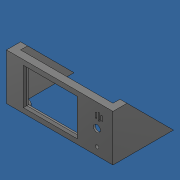
# Autodesk Inventor part: LCD_Holder
Saved by Autodesk Inventor 2020 (Build 240168000, 168)
## iProperties
Created: 2020-11-15
Part Number: LCD_Holder
Material: 一般
Document SubType Name: Modeling
Designer: kenta iguchi
Density: 1 g/cm^3
Appearance: 滑らか - 黒
Author: kenta iguchi
Autodesk Inventor part; units mm, degrees
ref_plane "YZ Plane" through (0, 0, 0) normal (1, 0, 0) x (0, 1, 0)
ref_plane "XZ Plane" through (0, 0, 0) normal (0, 1, 0) x (-1, 0, 0)
ref_plane "XY Plane" through (0, 0, 0) normal (0, 0, 1) x (1, 0, 0)
sketch "スケッチ1" plane through (0, 0, 0) normal (0, 0, 1) x (1, 0, 0)
  line L0 (18, -19) -> (-39.5, -19)
  line L1 (-39.5, -19) -> (-39.5, 19)
  line L2 (-39.5, 19) -> (18, 19)
  line L3 (18, 19) -> (18, -19)
  line L4 (18, -19) -> (-39.5, 19) construction
  line L5 (-39.5, -19) -> (18, 19) construction
  line L6 (-52.5, -23.5) -> (52.5, -23.5)
  line L7 (52.5, -23.5) -> (52.5, 23.5)
  line L8 (52.5, 23.5) -> (-52.5, 23.5)
  line L9 (-52.5, 23.5) -> (-52.5, -23.5)
  line L10 (-52.5, -23.5) -> (52.5, 23.5) construction
  line L11 (52.5, -23.5) -> (-52.5, 23.5) construction
  point P0 (0, 0)
  point P1 (0, 0)
  point P2 (-10.75, 0)
  point P3 (0, 0)
  dimension "d0" = 38
  dimension "d1" = 57.5
  dimension "d5" = 47
  dimension "d167" = 105
  dimension "d168" = 13
  constraints: 24 end point, 5 midpoint, 4 parallel, 2 horizontal, 2 perpendicular, 1 horizontal alignment, 1 other
  measures "d0" distance of L2.end L0.start
  measures "d1" distance of L0.start L0.end
  measures "d5" distance of L6.end L7.end
  measures "d167" distance of L6.start L6.end
  measures "d168" distance between parallel lines of L1 L9
extrude "押し出し1" add sketch "スケッチ1" against normal blind 4
sketch "スケッチ2" plane through (0, 0, 0) normal (0, 0, 1) x (1, 0, 0)
  line L0 (52.5, 23.5) -> (-52.5, 23.5) projected
  line L1 (-43.5, 20.5) -> (49.5, 20.5)
  line L2 (49.5, 20.5) -> (49.5, -20.5)
  line L3 (49.5, -20.5) -> (-43.5, -20.5)
  line L4 (-43.5, -20.5) -> (-43.5, 20.5)
  line L5 (-52.5, 23.5) -> (52.5, 23.5) projected
  line L6 (-52.5, 23.5) -> (-52.5, -23.5) projected
  point P0 (0, 0)
  point P1 (3, 20.5)
  dimension "d8" = 93
  dimension "d9" = 41
  dimension "d169" = 3
  dimension "d170" = 9
  constraints: 8 end point, 2 parallel, 1 horizontal, 1 midpoint, 1 perpendicular
  measures "d8" distance of L2.end L3.end
  measures "d9" distance of L1.end L2.end
  measures "d169" distance between parallel lines of L0 L1
  measures "d170" distance between parallel lines of L4 L6
hole "穴1" at (49.5, 20.5, 0) at (49.5, -20.5, 0) at (-43.5, -20.5, 0) at (-43.5, 20.5, 0) direction (0, 0, -1) diameter 4.3 depth 8 tip angle 118
sketch "スケッチ3" plane through (0, 0, 0) normal (0, 0, 1) x (1, 0, 0)
  line L0 (52.5, -23.5) -> (52.5, 23.5) projected
  circle A0 centre (42.65, -17.56) radius 2
  line L1 (-52.5, -23.5) -> (52.5, -23.5) projected
  point P0 (0, 0)
  dimension "d18" = 9.85
  dimension "d19" = 4
  dimension "d26" = 5.94
  constraints: 1 centre point, 1 coincident
  measures "d18" distance from line of point (42.65, -17.56) L0
  measures "d19" diameter of A0
  measures "d26" distance from line of point (42.65, -17.56) L1
extrude "押し出し2" cut sketch "スケッチ3" against normal blind 10
sketch "スケッチ4" plane through (0, 0, -4) normal (0, 0, -1) x (-1, 0, 0)
  circle A0 centre (-42.65, -17.56) radius 2 projected
  line L0 (-39.55, -14.46) -> (-45.75, -14.46)
  line L1 (-45.75, -14.46) -> (-45.75, -20.66)
  line L2 (-45.75, -20.66) -> (-39.55, -20.66)
  line L3 (-39.55, -20.66) -> (-39.55, -14.46)
  line L4 (-39.55, -14.46) -> (-45.75, -20.66) construction
  line L5 (-45.75, -14.46) -> (-39.55, -20.66) construction
  point P0 (0, 0)
  dimension "d22" = 6.2
  dimension "d23" = 6.2
  constraints: 12 end point, 2 midpoint, 2 parallel, 1 horizontal, 1 perpendicular
  measures "d22" distance of L2.end L1.end
  measures "d23" distance of L1.end L0.end
extrude "押し出し3" cut sketch "スケッチ4" against normal blind 1
sketch "スケッチ5" plane through (0, 0, 0) normal (0, 0, 1) x (1, 0, 0)
  circle A0 centre (42.37, 0.44) radius 4
  circle A1 centre (42.65, -17.56) radius 2 projected
  point P0 (0, 0)
  dimension "d29" = 8
  dimension "d171" = 18
  dimension "d172" = 0.28
  constraints: 1 centre point, 1 coincident
  measures "d29" diameter of A0
  measures "d171" vertical distance of A0.centre A1.centre
  measures "d172" horizontal distance of A1.centre A0.centre
extrude "押し出し4" cut sketch "スケッチ5" against normal through all contours A0
chamfer "面取り1" distance 2 angle 45 4 edges at (-39.5, 0, 0) (-10.75, 19, 0) (18, 0, 0) (-10.75, -19, 0)
sketch "スケッチ6" plane through (0, 0, -4) normal (0, 0, -1) x (-1, 0, 0)
  circle A0 centre (-42.37, 0.44) radius 4 projected
  line L0 (-48.87, -6.06) -> (-35.87, -6.06)
  line L1 (-35.87, -6.06) -> (-35.87, 6.94)
  line L2 (-35.87, 6.94) -> (-48.87, 6.94)
  line L3 (-48.87, 6.94) -> (-48.87, -6.06)
  line L4 (-48.87, -6.06) -> (-35.87, 6.94) construction
  line L5 (-35.87, -6.06) -> (-48.87, 6.94) construction
  point P0 (0, 0)
  dimension "d35" = 13
  dimension "d36" = 13
  constraints: 12 end point, 2 midpoint, 2 parallel, 1 horizontal, 1 perpendicular
  measures "d35" distance of L2.end L1.end
  measures "d36" distance of L1.end L0.end
extrude "押し出し5" cut sketch "スケッチ6" against normal blind 2
sketch "スケッチ7" plane through (0, 0, 0) normal (0, 0, 1) x (1, 0, 0)
  line L0 (52.5, 23.5) -> (-52.5, 23.5) projected
  line L1 (52.5, -23.5) -> (52.5, 23.5) projected
  circle A0 centre (44.69, 12.91) radius 4.5
  line L2 (44.69, 17.41) -> (44.69, 8.41) construction
  line L3 (43.94, 16.66) -> (43.94, 9.16)
  line L4 (45.44, 9.16) -> (45.44, 16.66)
  arc A1 (45.44, 16.66) -> (43.94, 16.66) centre (44.69, 16.66) ccw
  arc A2 (43.94, 9.16) -> (45.44, 9.16) centre (44.69, 9.16) ccw
  line L5 (41.69, 16.2641) -> (41.69, 9.5559) construction
  line L6 (40.94, 15.5141) -> (40.94, 10.3059)
  line L7 (42.44, 10.3059) -> (42.44, 15.5141)
  arc A3 (42.44, 15.5141) -> (40.94, 15.5141) centre (41.69, 15.5141) ccw
  arc A4 (40.94, 10.3059) -> (42.44, 10.3059) centre (41.69, 10.3059) ccw
  line L8 (47.69, 16.2641) -> (47.69, 9.5559) construction
  line L9 (46.94, 15.5141) -> (46.94, 10.3059)
  line L10 (48.44, 10.3059) -> (48.44, 15.5141)
  arc A5 (48.44, 15.5141) -> (46.94, 15.5141) centre (47.69, 15.5141) ccw
  arc A6 (46.94, 10.3059) -> (48.44, 10.3059) centre (47.69, 10.3059) ccw
  point P0 (0, 0)
  point P1 (41.69, 12.91)
  point P2 (47.69, 12.91)
  dimension "d39" = 7.81
  dimension "d40" = 10.59
  dimension "d41" = 9
  dimension "d42" = 1.5
  dimension "d43" = 1.5
  dimension "d44" = 1.5
  dimension "d45" = 3
  dimension "d46" = 6
  constraints: 24 end point, 24 point on circle, 12 tangent, 7 centre point, 6 point on line, 4 parallel, 3 midpoint, 2 coincident, 2 vertical
  measures "d39" distance from line of point (44.69, 12.91) L1
  measures "d40" distance from line of point (44.69, 12.91) L0
  measures "d41" diameter of A0
  measures "d42" diameter of A2
  measures "d43" diameter of A4
  measures "d44" diameter of A6
  measures "d45" distance of A0.centre point (41.69, 12.91)
  measures "d46" distance between parallel lines of L8 L5
extrude "押し出し6" cut sketch "スケッチ7" against normal blind 10 contours L10 A0 A6 L9 A5 | A0 A5 L10 | L10 A6 A0 | A1 L4 A2 L3 | A3 L7 A4 A0 L6 | A0 L6 A3 | A4 L6 A0
sketch "スケッチ8" plane through (0, 0, -4) normal (0, 0, -1) x (-1, 0, 0)
  line L0 (-46.94, 15.5141) -> (-46.94, 10.3059) projected
  arc A0 (-48.44, 10.3059) -> (-46.94, 10.3059) centre (-47.69, 10.3059) ccw projected
  line L1 (-48.44, 10.3059) -> (-48.44, 15.5141) projected
  arc A1 (-46.94, 15.5141) -> (-48.44, 15.5141) centre (-47.69, 15.5141) ccw projected
  line L2 (-45.44, 9.16) -> (-45.44, 16.66) projected
  arc A2 (-43.94, 16.66) -> (-45.44, 16.66) centre (-44.69, 16.66) ccw projected
  line L3 (-43.94, 16.66) -> (-43.94, 9.16) projected
  arc A3 (-45.44, 9.16) -> (-43.94, 9.16) centre (-44.69, 9.16) ccw projected
  line L4 (-40.94, 15.5141) -> (-40.94, 10.3059) projected
  arc A4 (-42.44, 10.3059) -> (-40.94, 10.3059) centre (-41.69, 10.3059) ccw projected
  line L5 (-42.44, 10.3059) -> (-42.44, 15.5141) projected
  arc A5 (-40.94, 15.5141) -> (-42.44, 15.5141) centre (-41.69, 15.5141) ccw projected
  line L6 (-44.69, 9.16) -> (-44.69, 16.66)
  circle A6 centre (-44.69, 12.91) radius 5
  point P0 (0, 0)
  dimension "d49" = 10
  constraints: 2 end point, 1 centre point, 1 coincident, 1 midpoint, 1 vertical
  measures "d49" diameter of A6
extrude "押し出し7" cut sketch "スケッチ8" against normal blind 2
sketch "スケッチ9" plane through (0, 0, 0) normal (0, 0, 1) x (1, 0, 0)
  line L0 (52.5, 23.5) -> (-52.5, 23.5) projected
  line L1 (-52.5, 23.5) -> (-52.5, -23.5) projected
  line L2 (-52.5, -23.5) -> (52.5, -23.5) projected
  line L3 (52.5, -23.5) -> (52.5, 23.5) projected
  line L4 (-55.5, 26.5) -> (55.5, 26.5)
  line L5 (55.5, 26.5) -> (55.5, -26.5)
  line L6 (55.5, -26.5) -> (-55.5, -26.5)
  line L7 (-55.5, -26.5) -> (-55.5, 26.5)
  circle A0 centre (49.5, 20.5) radius 2.15 projected
  circle A1 centre (49.5, 20.5) radius 4
  point P0 (0, 0)
  dimension "d52" = 3
  dimension "d67" = 8
  constraints: 8 end point, 1 centre point, 1 coincident, 3 other
  measures "d52" distance between parallel lines of L0 L4
  measures "d67" diameter of A1
extrude "押し出し8" add sketch "スケッチ9" against normal up to surface (4 mm away) contours L0 A1 | A1 L3 | L4 L5 L6 L7
sketch "スケッチ10" plane through (0, 0, -4) normal (0, 0, -1) x (-1, 0, 0)
  circle A0 centre (43.5, -20.5) radius 2.15 projected
  circle A1 centre (-49.5, 20.5) radius 2.15 projected
  circle A2 centre (43.5, 20.5) radius 2.15 projected
  circle A3 centre (-49.5, 20.5) radius 2.2
  circle A4 centre (43.5, 20.5) radius 2.2
  circle A5 centre (43.5, -20.5) radius 2.2
  circle A6 centre (-49.5, -20.5) radius 2.15 projected
  circle A7 centre (-49.5, -20.5) radius 2.2
  circle A8 centre (-49.5, 20.5) radius 2.15 projected
  circle A9 centre (-49.5, 20.5) radius 4
  circle A10 centre (43.5, 20.5) radius 4
  circle A11 centre (43.5, -20.5) radius 4
  circle A12 centre (-49.5, -20.5) radius 4
  point P0 (0, 0)
  dimension "d55" = 4.4
  dimension "d56" = 4.4
  dimension "d57" = 4.4
  dimension "d58" = 4.4
  dimension "d59" = 8
  dimension "d60" = 8
  dimension "d61" = 8
  dimension "d62" = 8
  constraints: 8 centre point, 8 coincident
  measures "d55" diameter of A3
  measures "d56" diameter of A4
  measures "d57" diameter of A5
  measures "d58" diameter of A7
  measures "d59" diameter of A9
  measures "d60" diameter of A10
  measures "d61" diameter of A11
  measures "d62" diameter of A12
extrude "押し出し9" add sketch "スケッチ10" along normal blind 3 contours A3 | A4 | A5 | A7 | A9 | A10 | A11 | A12
sketch "スケッチ11" plane through (0, 0, 0) normal (0, 0, 1) x (1, 0, 0)
  circle A0 centre (49.5, -20.5) radius 2.15 projected
  circle A1 centre (49.5, 20.5) radius 2.15 projected
  circle A2 centre (-43.5, -20.5) radius 2.15 projected
  circle A3 centre (-43.5, 20.5) radius 2.15 projected
  point P0 (0, 0)
extrude "押し出し10" add sketch "スケッチ11" against normal up to surface (4 mm away)
sketch "スケッチ12" plane through (0, 0, -4) normal (0, 0, -1) x (-1, 0, 0)
  circle A0 centre (43.5, 20.5) radius 4 projected
  arc A1 (-47.1508, 17.2625) -> (-47.5753, 16.9935) centre (-49.5, 20.5) ccw projected
  circle A2 centre (43.5, -20.5) radius 4 projected
  arc A3 (-45.75, -19.1081) -> (-45.5032, -20.66) centre (-49.5, -20.5) ccw projected
  line L0 (55.5, 26.5) -> (55.5, -26.5) projected
  line L1 (-55.5, 26.5) -> (55.5, 26.5) projected
  line L2 (-55.5, -26.5) -> (-55.5, 26.5) projected
  line L3 (55.5, -26.5) -> (-55.5, -26.5) projected
  line L4 (52.7, 23.7) -> (52.7, -23.7)
  line L5 (52.7, -23.7) -> (-52.7, -23.7)
  line L6 (-52.7, -23.7) -> (-52.7, 23.7)
  line L7 (-52.7, 23.7) -> (52.7, 23.7)
  circle A4 centre (-49.5, 20.5) radius 4 projected
  line L8 (-18, -19) -> (-18, 19) projected
  line L9 (-18, 19) -> (39.5, 19) projected
  line L10 (39.5, 19) -> (39.5, -19) projected
  line L11 (39.5, -19) -> (-18, -19) projected
  line L12 (-35.87, 6.94) -> (-35.87, -6.06) projected
  line L13 (-35.87, -6.06) -> (-48.87, -6.06) projected
  line L14 (-48.87, -6.06) -> (-48.87, 6.94) projected
  line L15 (-48.87, 6.94) -> (-35.87, 6.94) projected
  arc A5 (-47.1508, 17.2625) -> (-47.5753, 16.9935) centre (-49.5, 20.5) ccw projected
  arc A6 (-47.5753, 16.9935) -> (-47.1508, 17.2625) centre (-44.69, 12.91) ccw projected
  line L16 (55.5, -26.5) -> (-55.5, -26.5) projected
  line L17 (55.5, 26.5) -> (55.5, -26.5) projected
  line L18 (-55.5, 26.5) -> (55.5, 26.5) projected
  line L19 (-55.5, -26.5) -> (-55.5, 26.5) projected
  circle A7 centre (43.5, -20.5) radius 4 projected
  circle A8 centre (43.5, 20.5) radius 4 projected
  arc A9 (-45.75, -19.1081) -> (-45.5032, -20.66) centre (-49.5, -20.5) ccw projected
  line L20 (-45.75, -19.1081) -> (-45.75, -14.46) projected
  line L21 (-45.75, -14.46) -> (-39.55, -14.46) projected
  line L22 (-39.55, -14.46) -> (-39.55, -20.66) projected
  line L23 (-39.55, -20.66) -> (-45.5032, -20.66) projected
  point P0 (0, 0)
  point P1 (-47.1, 23.7)
  point P2 (41.1, 23.7)
  point P3 (52.7, 17.5876)
  point P4 (52.7, -17.5876)
  point P5 (41.1, -23.7)
  point P6 (-47.1, -23.7)
  point P7 (-52.7, -18.1)
  point P8 (-52.7, 18.1)
  point P9 (45.9, 23.7)
  point P10 (-51.9, 23.7)
  point P11 (-52.7, 22.9)
  point P12 (-52.7, -22.9)
  point P13 (-51.9, -23.7)
  point P14 (45.9, -23.7)
  dimension "d68" = 2.8
  constraints: 8 end point, 3 other
  measures "d68" distance between parallel lines of L1 L7
extrude "押し出し11" add sketch "スケッチ12" along normal blind 4 contours A1 L6 L7 | L5 L6 A3 | L0 L3 L2 L1
sketch "スケッチ14" plane through (0, 0, -8) normal (0, 0, -1) x (-1, 0, 0)
  line L0 (55.5, -26.5) -> (55.5, 26.5) projected
  line L1 (-52.7, -18.1) -> (-52.7, 18.1) projected
  line L2 (52.7, 23.7) -> (52.7, -23.7) projected
  line L3 (-55.5, 26.5) -> (55.5, 26.5) projected
  line L4 (55.5, 26.5) -> (60.7, 26.5)
  line L5 (60.7, 26.5) -> (60.7, -26.5)
  line L6 (60.7, -26.5) -> (55.5, -26.5)
  line L7 (55.5, -26.5) -> (55.5, 26.5)
  line L8 (-55.5, 26.5) -> (-60.7, 26.5)
  line L9 (-60.7, 26.5) -> (-60.7, -26.5)
  line L10 (-60.7, -26.5) -> (-55.5, -26.5)
  line L11 (-55.5, -26.5) -> (-55.5, 26.5)
  point P0 (0, 0)
  point P1 (55.5, -26.5)
  point P2 (55.5, 26)
  point P3 (55.5, -26)
  dimension "d80" = 8
  dimension "d81" = 8
  constraints: 16 end point, 4 parallel, 2 horizontal, 2 perpendicular, 1 horizontal alignment, 1 point on line
  measures "d80" distance between parallel lines of L5 L2
  measures "d81" distance between parallel lines of L9 L1
extrude "押し出し13" add sketch "スケッチ14" against normal up to surface (8 mm away)
sketch "スケッチ16" plane through (0, 0, -8) normal (0, 0, -1) x (-1, 0, 0)
  line L0 (-60.7, -26.5) -> (60.7, -26.5) projected
  line L1 (-60.7, 26.5) -> (-52.7, 26.5)
  line L2 (-52.7, 26.5) -> (-52.7, -26.5)
  line L3 (-52.7, -26.5) -> (-60.7, -26.5)
  line L4 (-60.7, -26.5) -> (-60.7, 26.5)
  line L5 (60.7, 26.5) -> (-60.7, 26.5) projected
  line L6 (60.7, 26.5) -> (52.7, 26.5)
  line L7 (52.7, 26.5) -> (52.7, -26.5)
  line L8 (52.7, -26.5) -> (60.7, -26.5)
  line L9 (60.7, -26.5) -> (60.7, 26.5)
  point P0 (-52.7, -18.1)
  point P1 (52.7, 17.5876)
  point P2 (0, 0)
  point P3 (60.7, -26.5)
  constraints: 16 end point, 4 parallel, 2 horizontal, 2 perpendicular, 2 point on line, 1 vertical alignment
extrude "押し出し14" add sketch "スケッチ16" along normal blind 10 contours L4 L1 L2 L0 | L7 L5 L9 L0
chamfer "面取り4" distance 2 angle 45 2 edges at (-56.7, 26.5, -18) (56.7, 26.5, -18)
sketch "スケッチ17" plane through (-60.7, -26.5, 0) normal (-1, 0, 0) x (0, 0, 1)
  line L0 (-18, 0) -> (-18, 51)
  line L1 (0, 0) -> (-8, 0)
  line L2 (-18, 51) -> (-69, 0)
  line L3 (-69, 0) -> (-18, 0)
  line L4 (0, 0) -> (-8, 0)
  line L5 (-18, 0) -> (-43.5, 25.5)
  line L6 (-18, 51) -> (-16, 53) projected
  line L7 (-18, 0) -> (-18, 51) projected
  line L8 (0, 0) -> (-18, 0) projected
  line L9 (0, 0) -> (0, 53) projected
  line L10 (0, 53) -> (-16, 53) projected
  line L11 (-18, 51) -> (-16, 53) projected
  point P0 (0, 26.5)
  constraints: 12 end point, 2 collinear, 1 midpoint
extrude "押し出し15" add sketch "スケッチ17" against normal up to surface (8 mm away) contours L5 L2 L0 | L3 L2 L5
sketch "スケッチ18" plane through (60.7, -26.5, 0) normal (1, 0, 0) x (0, 0, -1)
  line L0 (18, 50) -> (18, 0) projected
  line L1 (4, 2.8) -> (4, 50.2) projected
  line L2 (8, 50.2) -> (8, 53) projected
  line L3 (8, 0) -> (8, 2.8) projected
  line L4 (8, 0) -> (69, 0) projected
  line L5 (16, 53) -> (69, 0) projected
  line L6 (8, 53) -> (16, 53) projected
  line L7 (4, 50.2) -> (8, 50.2) projected
  line L8 (4, 2.8) -> (8, 2.8) projected
  point P0 (0, 26.5)
  point P1 (18, 50)
  point P2 (18, 0)
extrude "押し出し16" add sketch "スケッチ18" against normal up to surface (8 mm away)
sketch "スケッチ20" plane through (-60.7, -26.5, 0) normal (-1, 0, 0) x (0, 0, 1)
  line L0 (0, 0) -> (0, 53) projected
  line L1 (-8.05, 12) -> (-12.05, 12)
  line L2 (-12.05, 12) -> (-12.05, 40)
  line L3 (-12.05, 40) -> (-8.05, 40)
  line L4 (-8.05, 40) -> (-8.05, 12)
  line L5 (0, 30.94) -> (0, 22.94) projected
  point P0 (0, 26.5)
  point P1 (-12.05, 26)
  point P2 (-10.05, 40)
  dimension "d97" = 4
  dimension "d173" = 28
  dimension "d174" = 0.5
  dimension "d175" = 10.05
  constraints: 8 end point, 2 midpoint, 2 parallel, 1 horizontal, 1 perpendicular
  measures "d97" distance of L2.end L3.end
  measures "d173" distance of L1.end L2.end
  measures "d174" vertical distance of point (0, 26.5) point (-12.05, 26)
  measures "d175" distance from line of point (-10.05, 40) L0
extrude "押し出し18" cut sketch "スケッチ20" against normal blind 10
fillet "フィレット2" radius 1 4 edges at (-56.7, 13.5, -12.05) (-56.7, 13.5, -8.05) (-56.7, -14.5, -8.05) (-56.7, -14.5, -12.05)
sketch "スケッチ24" plane through (62.1, 26, -16) normal (0, 0.7071068, -0.7071068) x (-1, 0, 0)
  line L0 (0, 0) -> (0, -38.1838) projected
  line L1 (0, -38.1838) -> (-12, -38.1838)
  line L2 (-12, -38.1838) -> (-12, -18.1838)
  line L3 (-12, -18.1838) -> (0, -18.1838)
  line L4 (0, -18.1838) -> (0, -38.1838)
  line L5 (113.4, 0) -> (113.4, -38.1838) projected
  line L6 (121.4, -38.1838) -> (121.4, 0) projected
  line L7 (121.4, 0) -> (113.4, 0) projected
  line L8 (121.4, -38.1838) -> (121.4, 0) projected
  line L9 (121.4, -38.1838) -> (133.4, -38.1838)
  line L10 (133.4, -38.1838) -> (133.4, -18.1838)
  line L11 (133.4, -18.1838) -> (121.4, -18.1838)
  line L12 (121.4, -18.1838) -> (121.4, -38.1838)
  line L13 (121.4, -38.1838) -> (113.4, -38.1838) projected
  point P0 (62.1, -7.0711)
  point P1 (0, -18.1838)
  point P2 (8, -38.1838)
  dimension "d118" = 12
  dimension "d119" = 20
  dimension "d120" = 12
  dimension "d121" = 20
  constraints: 16 end point, 4 parallel, 2 horizontal, 2 horizontal alignment, 2 perpendicular
  measures "d118" distance of L2.end L3.end
  measures "d119" distance of L1.end L2.end
  measures "d120" distance of L11.end L10.end
  measures "d121" distance of L10.end L9.end
extrude "押し出し21" [suppressed]
chamfer "面取り6" [suppressed]
sketch "スケッチ26" plane through (51.44, 20.575, -18) normal (0, 0, 1) x (1, 0, 0)
  arc A0 (2.66, -2.9874) -> (2.66, 2.9874) centre (0, 0) ccw projected
  line L0 (2.66, 2.9874) -> (2.66, -2.9874) projected
  arc A1 (2.66, -44.1374) -> (2.66, -38.1626) centre (0, -41.15) ccw projected
  line L1 (2.66, -38.1626) -> (2.66, -44.1374) projected
  arc A2 (-102.74, 2.9874) -> (-102.74, -2.9874) centre (-100.08, 0) ccw projected
  line L2 (-102.74, -2.9874) -> (-102.74, 2.9874) projected
  arc A3 (-102.74, -38.1626) -> (-102.74, -44.1374) centre (-100.08, -41.15) ccw projected
  line L3 (-102.74, -44.1374) -> (-102.74, -38.1626) projected
  point P0 (-51.44, -20.575)
sketch "スケッチ27" plane through (0, 0, -8) normal (0, 0, -1) x (-1, 0, 0)
  line L0 (52.7, -26.5) -> (52.7, -23.5624) projected
  arc A0 (47.5431, -23.7) -> (52.7, -23.5624) centre (50.04, -20.575) ccw projected
  line L1 (47.5431, -23.7) -> (-47.5431, -23.7) projected
  arc A1 (-52.7, -23.5624) -> (-47.5431, -23.7) centre (-50.04, -20.575) ccw projected
  line L2 (-52.7, -26.5) -> (52.7, -26.5) projected
  line L3 (-52.7, -23.5624) -> (-52.7, -26.5) projected
  line L4 (52.7, 26) -> (55.5, 26) projected
  line L5 (55.5, 26) -> (55.5, 26.5) projected
  line L6 (55.5, 26.5) -> (-55.5, 26.5) projected
  line L7 (-55.5, 26.5) -> (-55.5, 26) projected
  line L8 (-55.5, 26) -> (-52.7, 26) projected
  line L9 (-52.7, 26) -> (-52.7, 23.5624) projected
  arc A2 (-47.5431, 23.7) -> (-52.7, 23.5624) centre (-50.04, 20.575) ccw projected
  line L10 (-47.5431, 23.7) -> (47.5431, 23.7) projected
  arc A3 (52.7, 23.5624) -> (47.5431, 23.7) centre (50.04, 20.575) ccw projected
  line L11 (52.7, 23.5624) -> (52.7, 26) projected
  point P0 (0, 0)
sketch "スケッチ29" plane through (-61.3, -1, -14.7157) normal (0, 0.7071068, -0.7071068) x (-1, 0, 0)
  arc A0 (8.5858, -0.5858) -> (7.1716, 0) centre (7.1716, -2) ccw projected
  line L0 (9.4142, -1.4142) -> (8.5858, -0.5858) projected
  arc A1 (10, -2.8284) -> (9.4142, -1.4142) centre (8, -2.8284) ccw projected
  line L1 (10, -2.8284) -> (10, -17.1716) projected
  arc A2 (9.4142, -18.5858) -> (10, -17.1716) centre (8, -17.1716) ccw projected
  line L2 (8.5858, -19.4142) -> (9.4142, -18.5858) projected
  arc A3 (7.1716, -20) -> (8.5858, -19.4142) centre (7.1716, -18) ccw projected
  line L3 (7.1716, -20) -> (-1.4142, -20) projected
  line L4 (-1.4142, -20) -> (-1.4142, 0.5858) projected
  arc A4 (-1.4142, 0.5858) -> (0, 0) centre (0, 2) ccw projected
  line L5 (0, 0) -> (7.1716, 0) projected
  arc A5 (-133.9858, -19.4142) -> (-132.5716, -20) centre (-132.5716, -18) ccw projected
  line L6 (-134.8142, -18.5858) -> (-133.9858, -19.4142) projected
  arc A6 (-135.4, -17.1716) -> (-134.8142, -18.5858) centre (-133.4, -17.1716) ccw projected
  line L7 (-135.4, -17.1716) -> (-135.4, -2.8284) projected
  arc A7 (-134.8142, -1.4142) -> (-135.4, -2.8284) centre (-133.4, -2.8284) ccw projected
  line L8 (-133.9858, -0.5858) -> (-134.8142, -1.4142) projected
  arc A8 (-132.5716, 0) -> (-133.9858, -0.5858) centre (-132.5716, -2) ccw projected
  line L9 (-132.5716, 0) -> (-125.4, 0) projected
  arc A9 (-125.4, 0) -> (-123.9858, 0.5858) centre (-125.4, 2) ccw projected
  line L10 (-123.9858, -20) -> (-123.9858, 0.5858) projected
  line L11 (-123.9858, -20) -> (-132.5716, -20) projected
  point P0 (-61.3, 11.1127)
  point P1 (-129.4, -10)
  point P2 (4, -10)
  dimension "d152" = 10
  dimension "d153" = 6
  dimension "d154" = 6
  constraints: 1 horizontal alignment
  measures "d152" distance from line of L11 point (-129.4, -10)
  measures "d153" distance from line of point (4, -10) L1
  measures "d154" distance from line of point (-129.4, -10) L7
sketch "スケッチ30" plane through (-61.3, -1, -14.7157) normal (0, 0.7071068, -0.7071068) x (-1, 0, 0)
  circle A0 centre (4, -10) radius 4 projected
  arc A1 (8.5858, -0.5858) -> (7.1716, 0) centre (7.1716, -2) ccw projected
  line L0 (9.4142, -1.4142) -> (8.5858, -0.5858) projected
  arc A2 (10, -2.8284) -> (9.4142, -1.4142) centre (8, -2.8284) ccw projected
  line L1 (10, -2.8284) -> (10, -17.1716) projected
  arc A3 (9.4142, -18.5858) -> (10, -17.1716) centre (8, -17.1716) ccw projected
  line L2 (8.5858, -19.4142) -> (9.4142, -18.5858) projected
  arc A4 (7.1716, -20) -> (8.5858, -19.4142) centre (7.1716, -18) ccw projected
  line L3 (7.1716, -20) -> (-1.4142, -20) projected
  line L4 (-1.4142, -20) -> (-1.4142, 0.5858) projected
  arc A5 (-1.4142, 0.5858) -> (0, 0) centre (0, 2) ccw projected
  line L5 (0, 0) -> (7.1716, 0) projected
  circle A6 centre (-129.4, -10) radius 4 projected
  arc A7 (-133.9858, -19.4142) -> (-132.5716, -20) centre (-132.5716, -18) ccw projected
  line L6 (-134.8142, -18.5858) -> (-133.9858, -19.4142) projected
  arc A8 (-135.4, -17.1716) -> (-134.8142, -18.5858) centre (-133.4, -17.1716) ccw projected
  line L7 (-135.4, -17.1716) -> (-135.4, -2.8284) projected
  arc A9 (-134.8142, -1.4142) -> (-135.4, -2.8284) centre (-133.4, -2.8284) ccw projected
  line L8 (-133.9858, -0.5858) -> (-134.8142, -1.4142) projected
  arc A10 (-132.5716, 0) -> (-133.9858, -0.5858) centre (-132.5716, -2) ccw projected
  line L9 (-132.5716, 0) -> (-125.4, 0) projected
  arc A11 (-125.4, 0) -> (-123.9858, 0.5858) centre (-125.4, 2) ccw projected
  line L10 (-123.9858, -20) -> (-123.9858, 0.5858) projected
  line L11 (-123.9858, -20) -> (-132.5716, -20) projected
  line L12 (17.8305, -6) -> (-146.9546, -6)
  line L13 (-146.9546, -6) -> (-146.9546, -14)
  line L14 (-146.9546, -14) -> (17.8305, -14)
  line L15 (17.8305, -14) -> (17.8305, -6)
  point P0 (-61.3, 11.1127)
  point P1 (-135.4, -14)
  point P2 (-129.4, -14)
  point P3 (-129.4, -6)
  point P4 (-135.4, -6)
  point P5 (4, -14)
  point P6 (10, -14)
  point P7 (10, -6)
  point P8 (4, -6)
  constraints: 8 end point, 2 parallel, 2 tangent, 1 horizontal, 1 perpendicular
